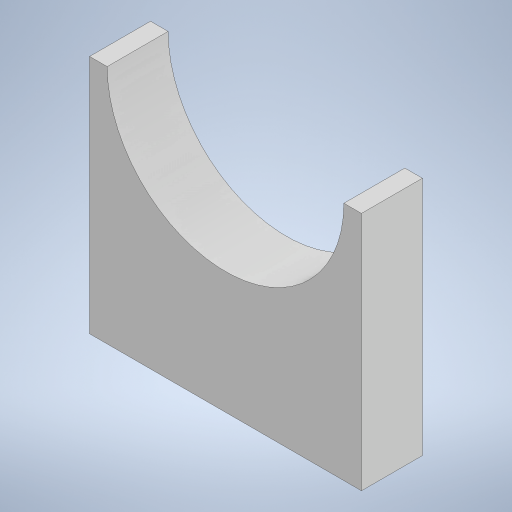
# Autodesk Inventor part: Button Cover
Saved by Autodesk Inventor 2023 (Build 270158000, 158)
## iProperties
Created: 2024-03-21
Part Number: Button Cover
Material: Generic
Document SubType Name: Modeling
Designer: Pobe Tran
Density: 1 g/cm^3
Appearance: Default
Author: Pobe Tran
Autodesk Inventor part; units mm, degrees
ref_plane "YZ Plane" through (0, 0, 0) normal (1, 0, 0) x (0, 1, 0)
ref_plane "XZ Plane" through (0, 0, 0) normal (0, 1, 0) x (-1, 0, 0)
ref_plane "XY Plane" through (0, 0, 0) normal (0, 0, 1) x (1, 0, 0)
sketch "Sketch6" plane through (0, 0, 0) normal (0, 0, 1) x (1, 0, 0)
  circle A0 centre (0, 0) radius 37
  line L0 (-42.5, 75.1) -> (42.5, 75.1)
  line L1 (42.5, 75.1) -> (42.5, -75.1)
  line L2 (42.5, -75.1) -> (-42.5, -75.1)
  line L3 (-42.5, -75.1) -> (-42.5, 75.1)
  line L4 (-42.5, 75.1) -> (42.5, -75.1) construction
  line L5 (42.5, 75.1) -> (-42.5, -75.1) construction
  line L6 (-42.5, 0) -> (42.5, 0)
  line L7 (-42.5, 0) -> (42.5, 0)
  point P0 (0, -37)
  point P1 (37, 0)
  point P2 (-37, 0)
  dimension "d25" = 74
  dimension "d26" = 85
  dimension "d27" = 38.1
  constraints: 16 end point, 4 midpoint, 2 horizontal, 2 parallel, 1 coincident, 1 perpendicular, 3 other
  measures "d26" distance of L0.start L0.end
  measures "d27" distance from line of L2 point (0, -37)
extrude "Extrusion5" add sketch "Sketch6" along normal blind 19.05 contours L6 L1 L2 L3 A0
body "Solid2"
